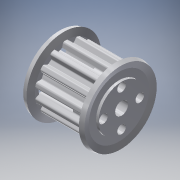
# Autodesk Inventor part: Timing Pulley - T5 4mm Bore 15mm Width
Saved by Autodesk Inventor 2017 SP1 (Build 210196100, 196)
## iProperties
Category: PARTsolutions
Company: MISUMI
Created: 2017-10-09
Part Number: Timing Pulley - T5 4mm Bore 15mm Width
Catalog Web Link: www.cadenas.de
Description: TTPA__T5100, TTPA__T5150, TTPA__T5200, TTPA__T5250, TTPB__T5100, TTPB__T5150, TTPB__T5200, TTPB__T5250, TTPK__T5100, TTPK__T5150, TTPK__T5200, TTPK__T5250, TTPN__T5100, TTPN__T5150, TTPN__T5200, TTPN__T5250, TTPT__T5100, TTPT__T5150, TTPT__T5200, TTPT__T5250, TTPM__T5100, TTPM__T5150, TTPM__T5200, TTPM__T5250, TTPP__T5100, TTPP__T5150, TTPP__T5200, TTPP__T5250_body-Timing Pulleys T5 Type
Vendor: MISUMI
Document SubType Name: Modeling
Designer: psAdmin
Manufacturer: MISUMI
Mass: 5.236 g
Surface Area: 40.3435 cm^2
Volume: 5.236 cm^3
Density: 1.06 g/cm^3
Material: ABS Plastic
Appearance: CR White
PSOL_IDENT_0: {$CADENAS_DATA\23d-libs\misumi\metric\51_timing_pulleys\ttpt_t5\ttpa_t5.prj},704 {VTYP=3D},{NB=TTPA1
PSOL_IDENT_1: 4T5150-A-C10_b},{LINA=TTPA14T5150-A-C10},{NN=TTPA__T5100, TTPA__T5150, TTPA__T5200, TTPA__T5250, TTP
PSOL_IDENT_2: B__T5100, TTPB__T5150, TTPB__T5200, TTPB__T5250, TTPK__T5100, TTPK__T5150, TTPK__T5200, TTPK__T5250,
PSOL_IDENT_3: TTPN__T5100, TTPN__T5150, TTPN__T5200, TTPN__T5250, TTPT__T5100, TTPT__T5150, TTPT__T5200, TTPT__T5
PSOL_IDENT_4: 250, TTPM__T5100, TTPM__T5150, TTPM__T5200, TTPM__T5250, TTPP__T5100, TTPP__T5150, TTPP__T5200, TTPP
PSOL_IDENT_5: __T5250_body},{DATE=27.04.2017 02:26:09},{GEOMDATE=25.07.2016 07:11:36},{VERSION=},{LINEID=320},{LIN
PSOL_IDENT_6: ESUBID=-1},{WBVAR=MATP,ST,TNW,PS,SBS,DD,Z,J,Q,R,S,T,ALT1,ALT2,M,QSC,QFC,QTC,ALT3,K,KSC,KFC,KTC,ALT4,
PSOL_IDENT_7: ZM,ZSC,ZFC,ZTC,ALT5,ALT6,ALT7,FC,ALT8,SRG,ALT9,BTC,TL,ALT10,TPC,ALT11,BC,ALT12,SLH}  {NB=TTPA14T5150
PSOL_IDENT_8: -A-C10_b},{LINA=TTPA14T5150-A-C10},{KT=DUMMY},{PN=TTPA14T5150-A-C10},{TYPE=TTPA},{MATP=A2017},{MATPA
PSOL_IDENT_9: LG= 'A2017','Aluminum Alloy 2000 series','S45C','1045 Carbon Steel Equivalent' },{ST=CA},{STALG= 'CA'
PSOL_IDENT_10: ,'Clear Anodize','BA','Black Anodize','HAT','Hard Clear Anodize','ENP','Electroless Nickel Plating'
PSOL_IDENT_11: },{NT=14},{TNW=T5150},{TNWALG= 'T5100','T5150','T5200','T5250' },{BW=15},{PS=A},{PSALG= 'A','B' },{S
PSOL_IDENT_12: BS=C},{SBSALG= 'H','Round Hole','P','Round Hole + Tap','N','New JIS Keywayed Bore + Tap (Standard)','
PSOL_IDENT_13: NK','New JIS Keywayed Bore + Tap (width 4.0mm, height 1.8mm)','C','Old JIS Keywayed Bore + Tap','V','
PSOL_IDENT_14: Stepped Hole','Y','Both Ends Stepped Hole','WB','Double Stepped Hole' },{DD=10.00},{DDALG=[10]},{DDH
PSOL_IDENT_15: A=[5:6/1],6.35,[7:12/1]},{DDPA=[5:6/1],6.35,[7:10/1]},{DDNA=[8:8/1],[10:10/1]},{DDCA=[10]},{DDVA=[5:
PSOL_IDENT_16: 6/1],6.35,[7:10/1]},{DDY=[5:10/1]},{DDWB=[5:8/1]},{DDHB=},{DDPB=},{DDNB=},{DDNK=[10:10/1]},{DDCB=},{
PSOL_IDENT_17: DDVFB=},{Z=0},{ZALG=[0]},{ZMIN=12.000},{ZAMAX=12.000},{ZBMAX=0.000},{DDZ=10.000},{J=0.0},{JALG=[0]},
PSOL_IDENT_18: {JMIN=2.000},{JMAX=20.000},{JPN=},{Q=0},{QALG=[0]},{QRMIN=12.000},{QRMAX=12.000},{WBQMIN=14.000},{R=
PSOL_IDENT_19: 0},{RALG=[0]},{WBRMAX=-2.000},{S=0.0},{SALG=[0]},{SMAX=14.000},{T=0.0},{TALG=[0]},{TMAX=14.000},{SBS
PSOL_IDENT_20: PN=-C10},{A=17},{W=22},{L=0},{PD=22.28},{OD=21.45},{D=0},{DALG=14.000},{DE=16.000},{F=26},{E=16},{TT=
PSOL_IDENT_21: 1.6},{BBK=4.000},{TTK=1.500},{ALT1=},{ALT1ALG= '','w/o KC90 (Set Screw Angle)','KC90','with KC90 (Se
PSOL_IDENT_22: t Screw Angle)' },{ANG=128.571},{ALT1PN=},{ALT2=},{ALT2ALG= '','Not applicable' },{M=N/A},{MALG= 'N/
PSOL_IDENT_23: A' },{MFTALG= 'N/A' },{MSALG= 'N/A' },{M3D=0.000},{KDML=0.000},{ML=0.000},{MUL=0.000},{PITCH=0.000},
PSOL_IDENT_24: {QSC=0.0},{QSCALG=0},{QFC=0.0},{QFCALG=0},{QTC=0.0},{QTCALG=0},{QPCDMIN=0.000},{QPCDMINALG=0.000},{Q
PSOL_IDENT_25: PCDMAX=12.000},{ALT2PN=},{TAP=0.000},{ALT3=},{ALT3ALG= '','Not applicable' },{K=0.0},{KALG=0},{KMIN=
PSOL_IDENT_26: 4.000},{KFTMAX=0.000},{KSMAX=0.000},{KSC=0.0},{KSCALG=0},{KFC=0.0},{KFCALG=0},{KTC=0.0},{KTCALG=0},{
PSOL_IDENT_27: KSCMIN=14.000},{KPCDMIN=14.000},{KPCDMAX=12.000},{ALT3PN=},{ALT4=},{ALT4ALG= '','Not applicable' },{
PSOL_IDENT_28: ALT4MIN=20.500},{ALT4MAX=5.500},{ZM=N/A},{ZMALG= 'N/A' },{ZMFTALG= 'N/A' },{ZMSALG= 'N/A' },{ZMDD1=0
PSOL_IDENT_29: .0},{ZMDD2=0.0},{ZMHH=0.0},{ZSC=0.0},{ZSCALG=[0]},{ZFC=0.0},{ZFCALG=[0]},{ZTC=0.0},{ZTCALG=[0]},{ZPC
PSOL_IDENT_30: DMIN=0.000},{ZPCDMINALG=0.000},{ZPCDMAX=12.000},{ALT4PN=},{ALT5=},{ALT5ALG= '','w/o Flange not Attac
PSOL_IDENT_31: hed','NFC','with NFC (Flange not Attached)' },{ALT5PN=},{ALT6=},{ALT6ALG= '','w/o Flange Attached on
PSOL_IDENT_32: One Side Only','RFC','with RFC (Flange Attached on The Boss Side Only)','LFC','with LFC (Flange Att
PSOL_IDENT_33: ached on The Opposite Side Only)' },{ALT6PN=},{ALT7=},{ALT7ALG= '','w/o FC (Flange Cut)','FC','with
PSOL_IDENT_34: FC (Flange Cut)' },{FC=0.0},{FCALG=0},{FCMIN=22.5},{FCMAX=24.0},{ALT7PN=},{ALT8=},{ALT8ALG= '','Not
PSOL_IDENT_35: applicable' },{ALT8ALGALG=12.000},{ALT8DD2=0.000},{ALT8MM=0.000},{ALT8NN=0.000},{QC=0.000},{KC=0.000
PSOL_IDENT_36: },{ZC=0.000},{SRG=0.0},{SRGALG=[0]},{SRGMAX=0.000},{DD2=0.0},{MM=0.00},{NN=0.00},{ALT8PN=},{ALT9=},{
PSOL_IDENT_37: ALT9ALG= '','Not applicable' },{BTC9=11.000},{TL9=1.000},{BTC=0},{BTCALG=[0]},{TL=0.0},{TLALG=0},{TL
PSOL_IDENT_38: MIN=1.000},{TLMAX=-22.500},{BTCL=0},{BTCD=0},{ALT9PN=},{WLBCTL=22.000},{ALT10=},{ALT10ALG= '','w/o T
PSOL_IDENT_39: PC (Tapped Hole Dimension)','TPC','with TPC (Tapped Hole Dimension)' },{TPC=N/A},{TPCALG= 'N/A' },{T
PSOL_IDENT_40: PCM=4.000},{ALT10PN=},{ALT11=},{ALT11ALG= '','Not applicable' },{BC=0.0},{BCALG=0},{BCMIN=7.000},{BC
PSOL_IDENT_41: MAX=-22.500},{M1WBC=11.000},{ALT11PN=},{KTT=4.225},{ALT12=},{ALT12ALG= '','w/o SLH (Set Screw Length
PSOL_IDENT_42: )','SLH','with SLH (Set Screw Length)' },{SLH=0},{SLHALG=[0]},{ALT12PN=},{AC=M4x3},{M1=4.000},{M1L=3
PSOL_IDENT_43: .000}
NN: TTPA__T5100, TTPA__T5150, TTPA__T5200, TTPA__T5250, TTPB__T5100, TTPB__T5150, TTPB__T5200, TTPB__T5250, TTPK__T5100, TTPK__T5150, TTPK__T5200, TTPK__T5250, TTPN__T5100, TTPN__T5150, TTPN__T5200, TTPN__T5250, TTPT__T5100, TTPT__T5150, TTPT__T5200, TTPT__T5250, TTPM__T5100, TTPM__T5150, TTPM__T5200, TTPM__T5250, TTPP__T5100, TTPP__T5150, TTPP__T5200, TTPP__T5250_body
NT: 14
NB: TTPA14T5150-A-C10_b
NBSYN: $PN._b
LINA: TTPA14T5150-A-C10
PN: TTPA14T5150-A-C10
MATP: Aluminum Alloy 2000 series
ST: Clear Anodize
TNW: T5150
BW: 15
PS: A
SBS: Old JIS Keywayed Bore + Tap
DD: 10.00
Z: 0
J: 0.0
Q: 0
R: 0
S: 0.0
T: 0.0
A: 17
W: 22
L: 0
PD: 22.28
OD: 21.45
F: 26
E: 16
ALT1: w/o KC90 (Set Screw Angle)
ALT2: Not applicable
M: N/A
QSC: 0.0
QFC: 0.0
QTC: 0.0
ALT3: Not applicable
K: 0.0
KSC: 0.0
KFC: 0.0
KTC: 0.0
ALT4: Not applicable
ZM: N/A
ZSC: 0.0
ZFC: 0.0
ZTC: 0.0
ALT5: w/o Flange not Attached
ALT6: w/o Flange Attached on One Side Only
ALT7: w/o FC (Flange Cut)
FC: 0.0
ALT8: Not applicable
SRG: 0.0
ALT9: Not applicable
BTC: 0
TL: 0.0
ALT10: w/o TPC (Tapped Hole Dimension)
TPC: N/A
ALT11: Not applicable
BC: 0.0
ALT12: w/o SLH (Set Screw Length)
SLH: 0
AC: M4x3
SUPPLIER: MISUMI
ARTICLENO: TTPA14T5150-A-C10_b
BOMINFO: TTPA14T5150-A-C10
CREATOR: CADENAS GmbH
Title: TTPA14T5150-A-C10
Author: Cadenas PARTsolutions
Comments: Timing Pulleys T5 Type
Autodesk Inventor part; units mm, degrees
ref_plane "YZ Plane" through (0, 0, 0) normal (1, 0, 0) x (0, 1, 0)
ref_plane "XZ Plane" through (0, 0, 0) normal (0, 1, 0) x (-1, 0, 0)
ref_plane "XY Plane" through (0, 0, 0) normal (0, 0, 1) x (1, 0, 0)
sketch "_____2" plane through (0, 0, 0) normal (0, 0, 1) x (1, 0, 0)
  line L0 (22, 0) -> (0, 0)
  line L1 (0, 0) -> (0, 8)
  line L2 (0, 8) -> (0.9, 8)
  line L3 (0.9, 8) -> (0.9, 10.5144)
  line L4 (0.9, 10.5144) -> (0.3449, 12.5859)
  line L5 (0.3449, 12.5859) -> (1.8904, 13)
  line L6 (1.8904, 13) -> (2.5, 10.725)
  line L7 (2.5, 10.725) -> (19.5, 10.725)
  line L8 (19.5, 10.725) -> (20.1096, 13)
  line L9 (20.1096, 13) -> (21.6551, 12.5859)
  line L10 (21.6551, 12.5859) -> (21.1, 10.5144)
  line L11 (21.1, 10.5144) -> (21.1, 8)
  line L12 (21.1, 8) -> (22, 8)
  line L13 (22, 8) -> (22, 0)
  line L14 (22, 0) -> (0, 0)
  constraints: 30 end point
revolve "Revolution1" add sketch "_____2" angle 360 about axis through (22, 0, 0) along (1, 0, 0)
sketch "Sketch2" plane through (22, 0, 0) normal (1, 0, 0) x (0, 0, -1)
  point P0 (0, 0)
hole "Hole1" at (22, 0, 0) direction (-1, 0, 0) diameter 4.5 depth 22
sketch "_____6" plane through (2.5, 0, 0) normal (1, 0, 0) x (0, 0, -1)
  line L0 (-2.0929, 10.9416) -> (-2.015, 10.534)
  arc A0 (-1.3585, 10.1983) -> (-2.015, 10.534) centre (-1.9022, 9.9447) ccw
  line L1 (-1.3585, 10.1983) -> (-0.8661, 9.1423)
  arc A1 (-0.8661, 9.1423) -> (-0.4819, 8.912) centre (-0.5035, 9.3114) ccw
  arc A2 (0.4819, 8.912) -> (-0.4819, 8.912) centre (0, 0) ccw
  arc A3 (0.4819, 8.912) -> (0.8661, 9.1423) centre (0.5035, 9.3114) ccw
  line L2 (0.8661, 9.1423) -> (1.3585, 10.1983)
  arc A4 (2.015, 10.534) -> (1.3585, 10.1983) centre (1.9022, 9.9447) ccw
  line L3 (2.015, 10.534) -> (2.0929, 10.9416)
  arc A5 (2.0929, 10.9416) -> (-2.0929, 10.9416) centre (0, 0) ccw
  constraints: 12 point on circle, 8 end point, 6 centre point
extrude "Extrusion1" cut sketch "_____6" along normal blind 17
pattern_circular "Circular Pattern1" count 14 over 360 about axis through (2.5, 0, 0) along (1, 0, 0) of "Extrusion1"
sketch "Sketch10" plane through (22, 0, 0) normal (1, 0, 0) x (0, 0, -1)
  circle A0 centre (0, -6.35) radius 1.5
  circle A1 centre (6.35, 0) radius 1.5
  circle A2 centre (0, 6.35) radius 1.5
  circle A3 centre (-6.35, 0) radius 1.5
  point P0 (0, 0)
  dimension "d40" = 3
  dimension "d41" = 6.35
  dimension "d44" = 360
  constraints: 4 centre point, 1 vertical alignment, 9 other
  measures "d40" diameter of A0
  measures "d41" distance of A0.centre point (0, 0)
extrude "Extrusion6" cut sketch "Sketch10" against normal through all
sketch "Sketch11" plane through (0, 0, 0) normal (-1, 0, 0) x (0, 0, 1)
  circle A0 centre (-6.35, 0) radius 1.5 projected
  circle A1 centre (-6.35, 0) radius 3
  circle A2 centre (0, -6.35) radius 3
  circle A3 centre (6.35, 0) radius 3
  circle A4 centre (0, 6.35) radius 3
  point P0 (0, 0)
  dimension "d48" = 6
  dimension "d51" = 360
  constraints: 4 centre point, 4 coincident, 13 other
  measures "d48" diameter of A1
extrude "Extrusion7" cut sketch "Sketch11" against normal blind 14 contours A0 | A1 | A2 | A3 | A4
body "Solid1"
